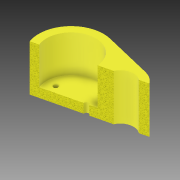
# Autodesk Inventor part: transducer_holder
Saved by Autodesk Inventor 2019 (Build 230136000, 136)
## iProperties
Created: 2019-01-04
Part Number: transducer_holder
Material: PC/ABS Plastic
Document SubType Name: Modeling
Designer: Callum Snowden
Mass: 1.66704 g
Surface Area: 32.7243 cm^2
Volume: 4.66602 cm^3
Density: 0.357273 g/cm^3
Appearance: Smooth - Yellow
Author: Callum Snowden
Autodesk Inventor part; units mm, degrees
ref_plane "YZ Plane" through (0, 0, 0) normal (1, 0, 0) x (0, 1, 0)
ref_plane "XZ Plane" through (0, 0, 0) normal (0, 1, 0) x (-1, 0, 0)
ref_plane "XY Plane" through (0, 0, 0) normal (0, 0, 1) x (1, 0, 0)
sketch "Sketch1" plane through (0, 0, 0) normal (0, 1, 0) x (-1, 0, 0)
  line L0 (0, -14.7) -> (0, 14.7) construction
  line L1 (-13.4, 0) -> (33.15, 0) construction
  circle A0 centre (0, 0) radius 4.25
  circle A1 centre (16, 0) radius 7.975
  arc A2 (13.5391, -10.2075) -> (13.5391, 10.2075) centre (16, 0) ccw
  arc A3 (-1.582, 6.562) -> (-1.582, -6.562) centre (0, 0) ccw
  line L2 (13.5391, 10.2075) -> (-1.582, 6.562)
  line L3 (13.5391, -10.2075) -> (-1.582, -6.562)
  circle A4 centre (21, 0) radius 0.75
  circle A5 centre (11, 0) radius 0.75
  line L4 (16, 7.975) -> (16, -7.975) construction
  dimension "d0" = 8.5
  dimension "d1" = 15.95
  dimension "d2" = 16
  dimension "d3" = 21
  dimension "d4" = 13.5
  dimension "d5" = 1.5
  dimension "d6" = 1.5
  dimension "d7" = 10
  constraints: 6 centre point, 6 end point, 6 point on circle, 4 tangent, 3 coincident, 3 point on line, 1 symmetric about line, 1 vertical
  measures "d0" diameter of A0
  measures "d1" diameter of A1
  measures "d2" distance of point (0, 0) A1.centre
  measures "d3" diameter of A2
  measures "d4" diameter of A3
  measures "d5" diameter of A4
  measures "d6" diameter of A5
  measures "d7" distance of A5.centre A4.centre
extrude "Base" add sketch "Sketch1" along normal blind 3 contours A1 | L3 A3 L2 A2
extrude "Walls" add sketch "Sketch1" along normal blind 15 contours L3 A3 L2 A2
equation "\"d6\" = d5"
body "Solid1"
